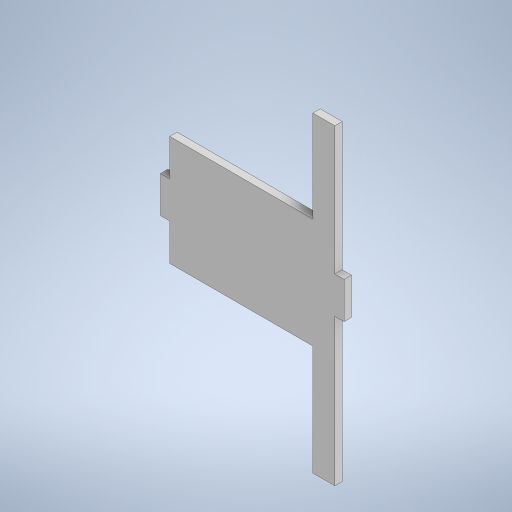
# Autodesk Inventor part: 外壳挡板
Saved by Autodesk Inventor 2023.1 (Build 271208000, 208)
## iProperties
Created: 2023-07-19
Part Number: 外壳挡板
Material: 常规
Document SubType Name: Modeling
Designer: Selcon
Density: 1 g/cm^3
Appearance: 默认
Author: Selcon
Autodesk Inventor part; units mm, degrees
ref_plane "YZ Plane" through (0, 0, 0) normal (1, 0, 0) x (0, 1, 0)
ref_plane "XZ Plane" through (0, 0, 0) normal (0, 1, 0) x (-1, 0, 0)
ref_plane "XY Plane" through (0, 0, 0) normal (0, 0, 1) x (1, 0, 0)
sketch "草图1" plane through (0, 0, 0) normal (0, 0, 1) x (1, 0, 0)
  line L0 (-30, 425) -> (30, 425)
  line L1 (30, 425) -> (30, -425)
  line L2 (30, -425) -> (-30, -425)
  line L3 (-30, -425) -> (-30, 425)
  line L4 (-510, 0) -> (120, 0) projected
  line L5 (0, -595) -> (0, 595) projected
  line L6 (-420, 175) -> (-30, 175)
  line L7 (-30, 175) -> (-30, -125)
  line L8 (-30, -125) -> (-420, -125)
  line L9 (-420, -125) -> (-420, 175)
  point P0 (0, 0)
  point P1 (-30, 175)
  dimension "d0" = 60
  dimension "d1" = 850
  dimension "d2" = 390
  dimension "d3" = 250
  dimension "d4" = 300
  constraints: 16 end point, 4 parallel, 2 horizontal, 2 perpendicular, 1 point on line, 2 other
  measures "d0" distance of L0.start L0.end
  measures "d1" distance of L0.end L1.end
  measures "d2" distance of L6.start L6.end
  measures "d3" distance between parallel lines of L6 L0
  measures "d4" distance of L8.end L6.start
extrude "拉伸1" add sketch "草图1" along normal mid plane 20
sketch "草图2" plane through (30, -425, 10) normal (1, 0, 0) x (0, 0, -1)
  line L0 (0, 0) -> (0, 850) projected
  line L1 (20, 850) -> (20, 0) projected
  line L2 (0, 500) -> (20, 500)
  line L3 (20, 500) -> (20, 400)
  line L4 (20, 400) -> (0, 400)
  line L5 (0, 400) -> (0, 500)
  line L6 (20, 850) -> (0, 850) projected
  point P0 (10, 425)
  point P1 (0, 400)
  dimension "d7" = 350
  dimension "d8" = 100
  constraints: 8 end point, 2 parallel, 2 point on line, 1 horizontal, 1 perpendicular
  measures "d7" distance between parallel lines of L6 L2
  measures "d8" distance between parallel lines of L4 L2
extrude "拉伸2" add sketch "草图2" along normal blind 25 contours L0 L2 L1 L4
sketch "草图3" plane through (-420, -125, 10) normal (-1, 0, 0) x (0, 0, 1)
  line L0 (-20, 0) -> (-20, 300) projected
  line L1 (0, 200) -> (0, 100) projected
  line L2 (-20, 200) -> (0, 200)
  line L3 (0, 200) -> (0, 100)
  line L4 (0, 100) -> (-20, 100)
  line L5 (-20, 100) -> (-20, 200)
  line L6 (-20, 550) -> (0, 550) projected
  point P0 (-10, 125)
  point P1 (-20, 100)
  point P2 (0, 200)
  dimension "d11" = 350
  dimension "d12" = 100
  constraints: 8 end point, 2 parallel, 2 point on line, 1 horizontal, 1 perpendicular
  measures "d11" distance between parallel lines of L6 L2
  measures "d12" distance between parallel lines of L4 L2
extrude "拉伸3" add sketch "草图3" along normal blind 25
